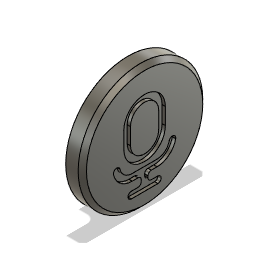
Record Button Cover v1 (Autodesk Fusion 360 design; units mm, degrees)
Autodesk Fusion 360 part; units mm, degrees
sketch "Sketch1" plane through (0, 0, 0) normal (1, 0, 0) x (0, 0, -1)
  circle A0 centre (0, 0) radius 4
  line L0 (2, 2) -> (-2, 2)
  line L1 (-2, 2) -> (-2, -2)
  line L2 (-2, -2) -> (2, -2)
  line L3 (2, -2) -> (2, 2)
  line L4 (2, 2) -> (-2, -2) construction
  line L5 (-2, 2) -> (2, -2) construction
  dimension "d1" = 8
  dimension "d2" = 4
  dimension "d3" = 4
  constraint coincident A0.centre origin
  constraint horizontal L0
  constraint perpendicular L0 L1
  constraint parallel L0 L2
  constraint parallel L1 L3
  constraint coincident L4 A0.centre
  constraint coincident L5 A0.centre
  measures "d1" diameter of A0
  measures "d2" distance of L0.start L0.end
  measures "d3" distance of L0.start L2.end
extrude "Extrude1" add sketch "Sketch1" along normal blind 2
sketch "Sketch2" plane through (2, 0, 0) normal (1, 0, 0) x (0, 0, -1)
  line L0 (2, 2) -> (2, -2)
  line L1 (2, -2) -> (-2, -2)
  line L2 (-2, -2) -> (-2, 2)
  line L3 (-2, 2) -> (2, 2)
  circle A0 centre (0, 0) radius 4
  circle A1 centre (0, 0) radius 7.5
  dimension "d6" = 15
  constraint coincident A0.centre A1.centre
  measures "d6" diameter of A1
extrude "Extrude2" add sketch "Sketch2" along normal blind 2 contours L0 L1 L2 L3 | A0 | A1
fillet "Fillet1" radius 1 1 edges at (2, -1.4465, 3.7293)
chamfer "Chamfer1" distance 0.5 angle 45 1 edges at (4, -2.7121, 6.9925)
sketch "Sketch3" plane through (4, 0, 0) normal (1, 0, 0) x (0, 0, -1)
  circle A0 centre (0, 0) radius 7
  line L0 (0, 0) -> (0, 2)
  line L1 (0, -4.8) -> (2, -4.8)
  line L2 (2, -4.8) -> (2, -5.6)
  line L3 (2, -5.6) -> (-2, -5.6)
  line L4 (-2, -5.6) -> (-2, -4.8)
  line L5 (0, -4.8) -> (-2, -4.8)
  line L6 (0, -3) -> (1.5, -3)
  line L7 (0, -3.8) -> (1.5, -3.8)
  line L8 (0, -3) -> (-1.5, -3)
  line L9 (0, -3.8) -> (-1.5, -3.8)
  line L10 (2.5, 2) -> (2.5, 0)
  line L11 (-2.5, 2) -> (-2.5, 0)
  line L12 (-1.7, 2) -> (-2.5, 2) construction
  line L13 (0, 2) -> (2.5, 2) construction
  line L14 (-1.7, 2) -> (-1.7, 0)
  line L15 (1.7, 2) -> (1.7, 0)
  arc A1 (-1.6925, 0.16) -> (1.6925, 0.16) centre (0, 0) ccw
  arc A2 (1.6925, 1.84) -> (-1.6925, 1.84) centre (0, 2) ccw
  arc A3 (-1.6925, 1.84) -> (-1.7, 1.833) centre (0, 0) ccw
  arc A4 (-1.7, 0.167) -> (-1.6925, 0.16) centre (0, 2) ccw
  arc A5 (-2.5, 0) -> (2.5, 0) centre (0, 0) ccw
  arc A6 (1.7, 1.833) -> (1.6925, 1.84) centre (0, 0) ccw
  arc A7 (1.6925, 0.16) -> (1.7, 0.167) centre (0, 2) ccw
  arc A8 (2.5, 2) -> (-2.5, 2) centre (0, 2) ccw
  line L16 (3, -1.5) -> (3.8, -1.5)
  arc A9 (1.5, -3) -> (3, -1.5) centre (1.5, -1.5) ccw
  arc A10 (1.5, -3.8) -> (3.8, -1.5) centre (1.5, -1.5) ccw
  line L17 (-3, -1.5) -> (-3.8, -1.5)
  arc A11 (-3.8, -1.5) -> (-1.5, -3.8) centre (-1.5, -1.5) ccw
  arc A12 (-3, -1.5) -> (-1.5, -3) centre (-1.5, -1.5) ccw
  line L18 (-0.4, -3.8) -> (0.4, -3.8)
  line L19 (0.4, -3.8) -> (0.4, -4.8)
  line L20 (0.4, -4.8) -> (-0.4, -4.8)
  line L21 (-0.4, -4.8) -> (-0.4, -3.8)
  dimension "d12" = 0.8
  dimension "d13" = 0.8
  dimension "d14" = 0.8
  dimension "d15" = 5
  dimension "d16" = 5
  dimension "d17" = 2
  dimension "d18" = 0.8
  dimension "d19" = 3
  dimension "d20" = 1.5
  dimension "d21" = 1.5
  dimension "d24" = 1.5
  dimension "d25" = 0.8
  dimension "d26" = 1.5
  dimension "d27" = 0.8
  dimension "d28" = 0.8
  dimension "d29" = 1.5
  dimension "d30" = 4
  dimension "d31" = 2
  dimension "d32" = 1
  dimension "d33" = 0.8
  dimension "d34" = 0.4
  constraint coincident A0.centre L0.start
  constraint concentric A1 A5
  constraint vertical L0
  constraint coincident L0.end L13.start
  constraint concentric A2 A4
  constraint perpendicular L1 L2
  constraint perpendicular L2 L3
  constraint perpendicular L3 L4
  constraint perpendicular L4 L5
  constraint coincident L10.start A4
  constraint vertical L10
  constraint vertical L11
  constraint horizontal L13
  constraint horizontal L12
  constraint coincident L12.start A2
  constraint coincident L14.end A1
  constraint tangent L14 A1
  constraint coincident L15.start A2
  constraint coincident L15.end A1
  constraint coincident L13 L15.start
  constraint horizontal A0.centre L15.end
  constraint horizontal A0.centre L14.end
  constraint coincident L14 A4.start
  constraint coincident L14 A3.end
  constraint coincident A2.end A5
  constraint concentric A3 A5
  constraint concentric A4 A7
  constraint coincident L15 A6.start
  constraint concentric A5 A6
  constraint coincident L15 A7.end
  constraint concentric A7 A8
  constraint vertical L6.end L7.end
  constraint vertical L8.end L9.end
  constraint vertical A0.centre L6.start
  constraint horizontal L6
  constraint horizontal L8
  constraint horizontal L9
  constraint vertical L6.end A9.centre
  constraint concentric A11 A12
  constraint horizontal L17
  constraint horizontal L18
  constraint vertical L19
  constraint horizontal L20
  constraint vertical L21
  constraint coincident L1 L19.end
  constraint coincident L9 L18.start
  measures "d12" distance of L1.end L2.end
  measures "d13" distance of A1 A5
  measures "d14" distance of A2 A4
  measures "d15" diameter of A4
  measures "d16" diameter of A5
  measures "d17" distance of A0.centre L0.end
  measures "d18" distance of L6 L7
  measures "d19" distance of L6 A0.centre
  measures "d20" distance of L6.start L6.end
  measures "d21" distance of L6.start L8.end
  measures "d24" distance of L6 L16
  measures "d25" distance of L16.start L16.end
  measures "d26" radius of A9
  measures "d27" distance of A11 A12
  measures "d28" distance of L17.end L17.start
  measures "d29" distance of L8 L17
  measures "d30" distance of L2.end L3.end
  measures "d31" distance of A0.centre L4
  measures "d32" distance of L1 L7
  measures "d33" distance of L19 L21
  measures "d34" distance of A0.centre L21
extrude "Extrude3" cut sketch "Sketch3" against normal blind 0.4 contours L1 L5 L7 L9 L18 L19 L20 L21 | L1 L2 L3 L4 L5 L20 | L6 L7 L8 L9 L16 A9 A10 L17 A11 A12 L18 | L10 L11 A5 A8
fillet "Fillet2" radius 0.4 12 edges at (3.8, -5.6, 2) (3.8, -4.8, 2) (3.8, -4.8, 0.4) (3.8, -3.8, 0.4) (3.8, -4.8, -2) (3.8, -5.6, -2) (3.8, -4.8, -0.4) (3.8, -3.8, -0.4) (3.8, -1.5, 3) (3.8, -1.5, 3.8) (3.8, -1.5, -3.8) (3.8, -1.5, -3)
